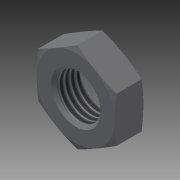
# Autodesk Inventor part: D-154
Saved by Autodesk Inventor 2014 (Build 180170000, 170)
## iProperties
Created: 2014-01-18
Part Number: D-154
Material: Steel
Catalog Web Link: www.cadenas.de
Description: Mounting Nut for Original Line Cylinders-
Vendor: BIMBA
Document SubType Name: Standard Catalog Part
Designer: Andrew Toennies
Manufacturer: BIMBA
Density: 1 g/cm^3
Appearance: Steel
Category: PARTsolutions
Company: BIMBA
PSOL_IDENT_0: {$CADENAS_DATA\23d-libs\bimba\bimba\bimba_imperial\bimba_full_line\original_line_cylinders\accessori
PSOL_IDENT_1: es\mounting_nut.prj},189 {VTYP=3D},{NB=D-154},{LINA=D-154},{NN=Mounting Nut for Original Line Cylind
PSOL_IDENT_2: ers},{DATE=11.06.2012 07:31:25},{GEOMDATE=10.11.2011 00:00:00},{VERSION=},{LINEID=40},{LINESUBID=-1}
PSOL_IDENT_3: ,{WBVAR=MAT}  {NB=D-154},{LINA=D-154},{KT=DUMMY},{PN=D-154},{PN1=D-154},{C=7/16-20},{TH=UNF},{MAT=},
PSOL_IDENT_4: {MAT1='','Zinc-Plated Carbon Steel', '-SS', 'Stainless Steel'},{A=0.69},{A1=0.69000000},{B=0.25},{B1=
PSOL_IDENT_5: 0.25000000},{NDM=0.43750000},{PITCH=0.0500},{DIA=-},{DIA2=-},{DIA3=-},{DIA1=0},{DIA4=0.00000000},{DI
PSOL_IDENT_6: A5=0.00000000},{T=-},{T2=-},{T3=-},{T1=0},{T4=0.00000000},{T5=0.00000000},{COLOR=0.75,0.75,0.75,0.00
PSOL_IDENT_7: },{TT=0.05000000},{TO=0.15000000},{PRA=1}
CNS_NN: Mounting Nut for Original Line Cylinders
CNS_NB: D-154
CNS_NBSYN: $PN.
CNS_LINA: D-154
CNS_PN: D-154
CNS_PN1: D-154
CNS_C: 7/16-20
CNS_TH: UNF
CNS_MAT: Zinc-Plated Carbon Steel
CNS_MAT1: '','Zinc-Plated Carbon Steel', '-SS', 'Stainless Steel'
CNS_A: 0.69
CNS_A1: 0.69000000
CNS_B: 0.25
CNS_B1: 0.25000000
CNS_NDM: 0.43750000
CNS_PITCH: 0.0500
CNS_DIA: -
CNS_DIA2: -
CNS_DIA3: -
CNS_DIA1: 0.000
CNS_DIA4: 0.00000000
CNS_DIA5: 0.00000000
CNS_T: -
CNS_T2: -
CNS_T3: -
CNS_T1: 0.000
CNS_T4: 0.00000000
CNS_T5: 0.00000000
CNS_COLOR: 0.75,0.75,0.75,0.00
CNS_TT: 0.05000000
CNS_TO: 0.15000000
CNS_PRA: 1
SUPPLIER: BIMBA
ARTICLENO: D-154
BOMINFO: D-154
CREATOR: CADENAS GmbH
Title: D-154
Author: Cadenas PARTsolutions
Autodesk Inventor part; units mm, degrees
ref_plane "YZ Plane" through (0, 0, 0) normal (1, 0, 0) x (0, 1, 0)
ref_plane "XZ Plane" through (0, 0, 0) normal (0, 1, 0) x (-1, 0, 0)
ref_plane "XY Plane" through (0, 0, 0) normal (0, 0, 1) x (1, 0, 0)
sketch "Sketch_8" plane through (0, 0, 0) normal (1, 0, 0) x (0, 1, 0)
  line L0 (0, -6.35) -> (0, 0)
  line L1 (0, 0) -> (8.763, 0)
  line L2 (8.763, 0) -> (10.5156, -0.4696)
  line L3 (10.5156, -0.4696) -> (10.5156, -5.8804)
  line L4 (10.5156, -5.8804) -> (8.763, -6.35)
  line L5 (8.763, -6.35) -> (0, -6.35)
  line L6 (0, -6.35) -> (0, 0)
  constraints: 14 end point
sketch "Sketch_10" plane through (0, 0, 0) normal (0, 0, 1) x (1, 0, 0)
  line L0 (-17.526, 17.526) -> (-17.526, -17.526)
  line L1 (-17.526, -17.526) -> (17.526, -17.526)
  line L2 (17.526, -17.526) -> (17.526, 17.526)
  line L3 (17.526, 17.526) -> (-17.526, 17.526)
  line L4 (-8.763, 5.0593) -> (-8.763, -5.0593)
  line L5 (-8.763, -5.0593) -> (0, -10.1186)
  line L6 (0, -10.1186) -> (8.763, -5.0593)
  line L7 (8.763, -5.0593) -> (8.763, 5.0593)
  line L8 (8.763, 5.0593) -> (0, 10.1186)
  line L9 (0, 10.1186) -> (-8.763, 5.0593)
  constraints: 20 end point
revolve "Revolution1" add sketch "Sketch_8" angle 360 about axis through (0, 0, -6.35) along (0, 0, -1)
extrude "Extrusion1" cut sketch "Sketch_10" against normal blind 6.35
sketch "Sketch_11" plane through (0, 0, 0) normal (1, 0, 0) x (0, 1, 0)
  line L0 (0, -6.35) -> (0, 0)
  line L1 (0, 0) -> (5.5563, 0)
  line L2 (5.5563, 0) -> (4.8692, -0.6871)
  line L3 (4.8692, -0.6871) -> (4.8692, -5.6629)
  line L4 (4.8692, -5.6629) -> (5.5563, -6.35)
  line L5 (5.5563, -6.35) -> (0, -6.35)
  line L6 (0, -6.35) -> (0, 0)
  constraints: 14 end point
revolve "Revolution2" cut sketch "Sketch_11" angle 360 about axis through (0, 0, -6.35) along (0, 0, -1)
thread "Thread1" size "7/16-20 UNF" class "2B" standard "ANSI Unified Screw Threads" full length
ref_plane "NUT_XY" through (0, 0, 0) normal (0, 0, 1) x (1, 0, 0)
ref_plane "NUT_YZ" through (0, 0, 0) normal (1, 0, 0) x (0, 1, 0)
ref_plane "NUT_ZX" through (0, 0, 0) normal (0, 1, 0) x (0, 0, 1)
ref_plane "a1_XY" through (-8.763, 8.763, 0) normal (0, 0, 1) x (1, 0, 0)
ref_plane "a1_YZ" through (-8.763, 8.763, 0) normal (1, 0, 0) x (0, 1, 0)
ref_plane "a1_ZX" through (-8.763, 8.763, 0) normal (0, 1, 0) x (0, 0, 1)
ref_plane "a2_XY" through (8.763, 8.763, 0) normal (0, 0, 1) x (1, 0, 0)
ref_plane "a2_YZ" through (8.763, 8.763, 0) normal (1, 0, 0) x (0, 1, 0)
ref_plane "a2_ZX" through (8.763, 8.763, 0) normal (0, 1, 0) x (0, 0, 1)
ref_plane "b1_XY" through (0, 8.763, 0) normal (1, 0, 0) x (0, 0, -1)
ref_plane "b1_YZ" through (0, 8.763, 0) normal (0, 0, -1) x (0, 1, 0)
ref_plane "b1_ZX" through (0, 8.763, 0) normal (0, 1, 0) x (1, 0, 0)
ref_plane "b2_XY" through (0, 8.763, -6.35) normal (1, 0, 0) x (0, 0, -1)
ref_plane "b2_YZ" through (0, 8.763, -6.35) normal (0, 0, -1) x (0, 1, 0)
ref_plane "b2_ZX" through (0, 8.763, -6.35) normal (0, 1, 0) x (1, 0, 0)
ref_plane "e_XY" through (0, 0, -6.35) normal (1, 0, 0) x (0, 0, -1)
ref_plane "e_YZ" through (0, 0, -6.35) normal (0, 0, -1) x (0, 1, 0)
ref_plane "e_ZX" through (0, 0, -6.35) normal (0, 1, 0) x (1, 0, 0)
ref_plane "ol1_XY" through (0, 0, -8.763) normal (0, 1, 0) x (1, 0, 0)
ref_plane "ol1_YZ" through (0, 0, -8.763) normal (1, 0, 0) x (0, 0, -1)
ref_plane "ol1_ZX" through (0, 0, -8.763) normal (0, 0, -1) x (0, 1, 0)
ref_plane "ol2_XY" through (6.35, 0, -8.763) normal (0, 1, 0) x (1, 0, 0)
ref_plane "ol2_YZ" through (6.35, 0, -8.763) normal (1, 0, 0) x (0, 0, -1)
ref_plane "ol2_ZX" through (6.35, 0, -8.763) normal (0, 0, -1) x (0, 1, 0)
ref_plane "th1_XY" through (0, 5.5563, -6.35) normal (1, 0, 0) x (0, 0, -1)
ref_plane "th1_YZ" through (0, 5.5563, -6.35) normal (0, 0, -1) x (0, 1, 0)
ref_plane "th1_ZX" through (0, 5.5563, -6.35) normal (0, 1, 0) x (1, 0, 0)
ref_plane "th2_XY" through (0, -5.5563, -6.35) normal (1, 0, 0) x (0, 0, -1)
ref_plane "th2_YZ" through (0, -5.5563, -6.35) normal (0, 0, -1) x (0, 1, 0)
ref_plane "th2_ZX" through (0, -5.5563, -6.35) normal (0, 1, 0) x (1, 0, 0)
body "Solid1"
